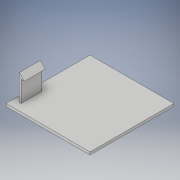
# Autodesk Inventor part: clip12_5
Saved by Autodesk Inventor 2019 (Build 230136000, 136)
## iProperties
Created: 2019-01-17
Part Number: clip12_5
Material: Generic
Document SubType Name: Modeling
Designer: assman
Density: 1 g/cm^3
Appearance: Default
Author: assman
Autodesk Inventor part; units mm, degrees
ref_plane "YZ Plane" through (0, 0, 0) normal (1, 0, 0) x (0, 1, 0)
ref_plane "XZ Plane" through (0, 0, 0) normal (0, 1, 0) x (-1, 0, 0)
ref_plane "XY Plane" through (0, 0, 0) normal (0, 0, 1) x (1, 0, 0)
sketch "Sketch1" plane through (0, 0, 0) normal (0, 0, 1) x (1, 0, 0)
  line L0 (0, 0) -> (-1, 0)
  line L1 (-1, 0) -> (-1, 12.5)
  line L2 (0, 0) -> (0, 9.9348)
  line L3 (0, 9.9348) -> (0, 12.5)
  line L4 (0, 12.5) -> (2, 12.5)
  line L5 (-1, 12.5) -> (-1, 15.5)
  line L6 (2, 12.5) -> (-1, 15.5)
  dimension "d0" = 1
  dimension "d4" = 12.5
  dimension "d6" = 2
  dimension "d7" = 45
  constraints: 14 end point, 3 vertical, 2 perpendicular, 1 horizontal
  measures "d0" distance of L0.start L0.end
  measures "d4" distance between parallel lines of L0 L4
  measures "d6" distance of L4.end L3.end
  measures "d7" angle of L5 L6
extrude "Extrusion1" add sketch "Sketch1" along normal blind 12.5
sketch "Sketch2" plane through (-1, 0, 0) normal (0, -1, 0) x (1, 0, 0)
  line L0 (-3.4473, 16.9327) -> (46.5527, 16.9327)
  line L1 (46.5527, 16.9327) -> (46.5527, -33.0673)
  line L2 (46.5527, -33.0673) -> (-3.4473, -33.0673)
  line L3 (-3.4473, -33.0673) -> (-3.4473, 16.9327)
  point P0 (1, 0)
  dimension "d10" = 50
  dimension "d11" = 50
  constraints: 8 end point, 2 parallel, 1 horizontal, 1 perpendicular
  measures "d10" distance of L1.end L2.end
  measures "d11" distance of L0.end L1.end
extrude "Extrusion2" add sketch "Sketch2" along normal blind 1.6 separate body
body "Solid1"
body "Solid2"
